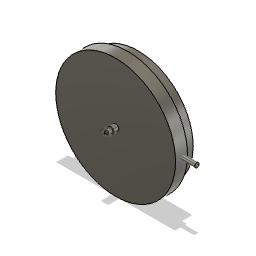
watch-model5 (Autodesk Fusion 360 archive; units mm, degrees)
design "movement-seiko-nh35"
Autodesk Fusion 360 part; units mm, degrees
sketch "Sketch1" plane through (0, 0, 0) normal (0, 0, 1) x (1, 0, 0)
  circle A0 centre (0, 0) radius 14.68
  dimension "d1" = 29.36
  constraint coincident A0.centre origin
  measures "d1" diameter of A0
extrude "Extrude1" add sketch "Sketch1" against normal blind 2.94 makes body 1
sketch "Sketch2" plane through (0, 0, -2.94) normal (0, 0, -1) x (-1, 0, 0)
  circle A0 centre (0, 0) radius 14.68
  circle A1 centre (0, 0) radius 13.5
  dimension "d4" = 27
  constraint coincident A0.centre A1.centre
  measures "d4" diameter of A1
extrude "Extrude2" add sketch "Sketch2" along normal blind 2.56 contours A1 bodies 1
sketch "Sketch3" plane through (0, 0, 0) normal (0, 0, 1) x (1, 0, 0)
  circle A0 centre (0, 0) radius 14.68
  circle A1 centre (0, 0) radius 0.75
  dimension "d7" = 1.5
  constraint concentric A0 A1
  measures "d7" diameter of A1
extrude "Extrude3" add sketch "Sketch3" along normal blind 1.18 contours A1 bodies 1
sketch "Sketch4" plane through (0, 0, 1.18) normal (0, 0, 1) x (1, 0, 0)
  circle A0 centre (0, 0) radius 0.75
  circle A1 centre (0, 0) radius 0.445
  dimension "d10" = 0.89
  constraint coincident A0.centre A1.centre
  measures "d10" diameter of A1
extrude "Extrude4" add sketch "Sketch4" along normal blind 0.99 contours A1 bodies 1
sketch "Sketch5" plane through (0, 0, 2.17) normal (0, 0, 1) x (1, 0, 0)
  circle A0 centre (0, 0) radius 0.445
  circle A1 centre (0, 0) radius 0.105
  dimension "d13" = 0.21
  constraint concentric A0 A1
  measures "d13" diameter of A1
extrude "Extrude5" add sketch "Sketch5" along normal blind 0.54 contours A1 bodies 1
sketch "Sketch6" plane through (0, 0, 0) normal (0, 0, 1) x (1, 0, 0)
  circle A0 centre (0, 0) radius 0.75
  circle A1 centre (0, 0) radius 14.68
  circle A2 centre (0, 0) radius 1
  dimension "d16" = 2
  constraint coincident A0.centre A1.centre
  measures "d16" diameter of A2
extrude "Extrude6" add sketch "Sketch6" along normal blind 2.76 separate body contours A2 makes body 2
sketch "Sketch7" plane through (0, 0, 0) normal (1, 0, 0) x (0, 0, -1)
  line L0 (0, 0) -> (1.92, 0) construction
  circle A0 centre (1.92, 0) radius 0.55
  dimension "d19" = 1.92
  dimension "d20" = 1.1
  constraint coincident L0.start origin
  constraint horizontal L0
  constraint coincident L0.end A0.centre
  measures "d19" distance of L0.start L0.end
  measures "d20" diameter of A0
extrude "Extrude7" add sketch "Sketch7" along normal blind 18 separate body makes body 3
equation "d5 = 5.5 mm - 2.94 mm"
equation "d8 = 0.4 mm + 0.78 mm"
equation "d11 = 0.4 mm + 1.37 mm - 0.78 mm"
equation "d14 = 1.91 mm - 1.37 mm"
equation "d17 = 0.4 mm + 1.91 mm + 0.45 mm"
named bodies: "to-crystal", "stem"
